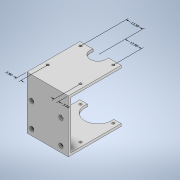
# Autodesk Inventor part: サーボモータ固定用
Saved by Autodesk Inventor 2022 (Build 260153000, 153)
## iProperties
Created: 2022-11-22
Part Number: サーボモータ固定用
Material: 一般
Document SubType Name: Modeling
Designer: tdn82
Density: 1 g/cm^3
Appearance: 既定
Author: tdn82
Autodesk Inventor part; units mm, degrees
ref_plane "YZ Plane" through (0, 0, 0) normal (1, 0, 0) x (0, 1, 0)
ref_plane "XZ Plane" through (0, 0, 0) normal (0, 1, 0) x (-1, 0, 0)
ref_plane "XY Plane" through (0, 0, 0) normal (0, 0, 1) x (1, 0, 0)
sketch "スケッチ1" plane through (0, 0, 0) normal (0, 1, 0) x (-1, 0, 0)
  line L0 (0, 0) -> (-34, 0)
  line L1 (-34, 0) -> (-34, -43.5)
  line L2 (-34, -43.5) -> (0, -43.5)
  line L3 (0, -43.5) -> (0, 0)
  dimension "d0" = 43.5
  dimension "d1" = 34
  constraints: 8 end point, 2 parallel, 1 horizontal, 1 perpendicular
  measures "d0" distance of L2.end L0.start
  measures "d1" distance of L0.start L0.end
extrude "押し出し1" add sketch "スケッチ1" along normal blind 43.5
sketch "スケッチ2" plane through (34, 0, 0) normal (1, 0, 0) x (0, 0, -1)
  line L0 (2, 41.5) -> (52, 41.5)
  line L1 (52, 41.5) -> (52, 2)
  line L2 (52, 2) -> (2, 2)
  line L3 (2, 2) -> (2, 41.5)
  line L4 (0, 43.5) -> (43.5, 43.5) projected
  line L5 (0, 0) -> (0, 43.5) projected
  dimension "d4" = 2
  dimension "d5" = 2
  dimension "d6" = 39.5
  dimension "d7" = 50
  constraints: 8 end point, 2 parallel, 1 horizontal, 1 perpendicular
  measures "d4" distance between parallel lines of L0 L4
  measures "d5" distance between parallel lines of L5 L3
  measures "d6" distance of L2.end L0.start
  measures "d7" distance of L0.start L0.end
extrude "押し出し2" cut sketch "スケッチ2" against normal blind 43.5
sketch "スケッチ3" plane through (0, 0, 0) normal (0, -1, 0) x (1, 0, 0)
  circle A0 centre (17, -41.5) radius 11
  line L0 (34, -43.5) -> (0, -43.5) projected
  line L1 (0, -43.5) -> (0, 0) projected
  point P0 (6.1833, -43.5)
  point P1 (27.8167, -43.5)
  dimension "d10" = 22
  dimension "d11" = 2
  dimension "d12" = 17
  constraints: 1 centre point
  measures "d10" diameter of A0
  measures "d11" distance from line of A0.centre L0
  measures "d12" distance from line of L1 A0.centre
extrude "押し出し3" cut sketch "スケッチ3" against normal blind 2 contours A0 L0 picked at (20.7405, -37.2254)
sketch "スケッチ4" plane through (0, 43.5, 0) normal (0, 1, 0) x (1, 0, 0)
  circle A0 centre (17, 41.5) radius 6.5
  line L0 (34, 43.5) -> (0, 43.5) projected
  line L1 (0, 43.5) -> (0, 0) projected
  point P0 (23.1847, 43.5)
  point P1 (10.8153, 43.5)
  point P2 (0, 35.0774)
  dimension "d15" = 13
  dimension "d16" = 2
  dimension "d17" = 17
  constraints: 1 centre point
  measures "d15" diameter of A0
  measures "d16" distance from line of L0 A0.centre
  measures "d17" distance from line of A0.centre L1
extrude "押し出し4" cut sketch "スケッチ4" against normal blind 2
sketch "スケッチ5" plane through (0, 43.5, 0) normal (0, 1, 0) x (1, 0, 0)
  line L0 (0, 0) -> (34, 0) projected
  line L1 (0, 43.5) -> (0, 0) projected
  line L2 (34, 0) -> (34, 43.5) projected
  point P0 (3.5, 13.5)
  point P1 (3.5, 40.5)
  point P2 (30.5, 40.5)
  point P3 (30.5, 13.5)
  dimension "d20" = 13.5
  dimension "d21" = 3.5
  dimension "d22" = 27
  dimension "d23" = 3.5
  dimension "d48" = 3.5
  measures "d20" distance from line of L0 point (3.5, 13.5)
  measures "d21" distance from line of point (3.5, 13.5) L1
  measures "d22" distance of point (3.5, 40.5) point (3.5, 13.5)
  measures "d23" distance from line of L2 point (30.5, 40.5)
  measures "d48" distance from line of point (30.5, 13.5) L2
hole "穴1" at (3.5, 43.5, -13.5) at (3.5, 43.5, -40.5) at (30.5, 43.5, -40.5) at (30.5, 43.5, -13.5) direction (0, -1, 0) diameter 2 end through all
sketch "スケッチ6" plane through (0, 0, 0) normal (0, 0, 1) x (1, 0, 0)
  line L0 (0, 0) -> (34, 0) projected
  line L1 (0, 0) -> (0, 43.5) projected
  point P0 (4, 5)
  point P1 (4, 25)
  point P2 (28, 5)
  point P3 (28, 25)
  dimension "d31" = 5
  dimension "d32" = 4
  dimension "d35" = 20
  dimension "d38" = 24
  constraints: 1 horizontal, 1 vertical, 3 other
  measures "d31" distance from line of L0 point (4, 5)
  measures "d32" distance from line of point (4, 5) L1
  measures "d35" distance of point (4, 5) point (4, 25)
  measures "d38" distance of point (4, 5) point (28, 5)
hole "穴2" at (4, 5, 0) at (4, 25, 0) at (28, 5, 0) at (28, 25, 0) direction (0, 0, -1) diameter 3.5 end through all
